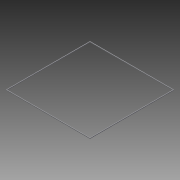
# Autodesk Inventor part: Outer Rim
Saved by Autodesk Inventor 2015 SP1 (Build 190203100, 203)
## iProperties
Created: 2015-06-11
Part Number: Outer Rim
Material: Generic
Document SubType Name: Modeling
Designer: Nathan
Density: 1 g/cm^3
Appearance: Default
Author: Nathan
Autodesk Inventor part; units mm, degrees
ref_plane "YZ Plane" through (0, 0, 0) normal (1, 0, 0) x (0, 1, 0)
ref_plane "XZ Plane" through (0, 0, 0) normal (0, 1, 0) x (-1, 0, 0)
ref_plane "XY Plane" through (0, 0, 0) normal (0, 0, 1) x (1, 0, 0)
sketch "Sketch1" plane through (0, 0, 0) normal (1, 0, 0) x (0, 1, 0)
  line L0 (-180, 180) -> (180, 180)
  line L1 (180, 180) -> (180, -180)
  line L2 (180, -180) -> (-180, -180)
  line L3 (-180, -180) -> (-180, 180)
  line L4 (-180, 180) -> (180, -180) construction
  line L5 (180, 180) -> (-180, -180) construction
  line L6 (-182.5, 182.5) -> (182.5, 182.5)
  line L7 (182.5, 182.5) -> (182.5, -182.5)
  line L8 (182.5, -182.5) -> (-182.5, -182.5)
  line L9 (-182.5, -182.5) -> (-182.5, 182.5)
  line L10 (-182.5, 182.5) -> (182.5, -182.5) construction
  line L11 (182.5, 182.5) -> (-182.5, -182.5) construction
  point P0 (0, 0)
  dimension "d0" = 360
  dimension "d1" = 360
  dimension "d2" = 365
  dimension "d3" = 365
  constraints: 24 end point, 4 midpoint, 4 parallel, 2 horizontal, 2 perpendicular
  measures "d0" distance of L1.end L2.end
  measures "d1" distance of L0.end L1.end
  measures "d2" distance of L7.end L8.end
  measures "d3" distance of L6.end L7.end
extrude "Extrusion1" add sketch "Sketch1" along normal blind 2.6
body "Solid1"
